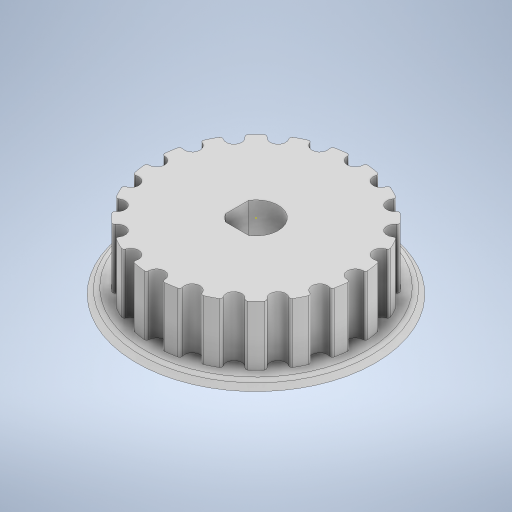
# Autodesk Inventor part: MuftaForRemenSmall
Saved by Autodesk Inventor 2024 (Build 280153000, 153)
## iProperties
Created: 2023-11-07
Part Number: MuftaForRemenSmall
Material: Generic
Document SubType Name: Modeling
Designer: KirikDK
Density: 1 g/cm^3
Appearance: Default
Author: KirikDK
Autodesk Inventor part; units mm, degrees
ref_plane "YZ Plane" through (0, 0, 0) normal (1, 0, 0) x (0, 1, 0)
ref_plane "XZ Plane" through (0, 0, 0) normal (0, 1, 0) x (-1, 0, 0)
ref_plane "XY Plane" through (0, 0, 0) normal (0, 0, 1) x (1, 0, 0)
sketch "Sketch1" plane through (0, 0, 0) normal (0, 1, 0) x (-1, 0, 0)
  circle A0 centre (0, 0) radius 32.5
  dimension "d0" = 65
  constraints: 1 centre point, 1 coincident
  measures "d0" diameter of A0
extrude "Extrusion1" add sketch "Sketch1" along normal blind 21
sketch "Sketch2" plane through (0, 0, 0) normal (0, -1, 0) x (1, 0, 0)
  circle A0 centre (0, 0) radius 38
  dimension "d5" = 76
  constraints: 1 centre point, 1 coincident
  measures "d5" diameter of A0
extrude "Extrusion2" add sketch "Sketch2" against normal blind 2
chamfer "Chamfer1" distance 2 angle 45 1 edges at (-38, 2, 0)
fillet "Fillet1" radius 2 1 edges at (-36.0001, 2, 0)
sketch "Sketch3" plane through (0, 21, 0) normal (0, 1, 0) x (1, 0, 0)
  circle A0 centre (0, 0) radius 7.05
  line L0 (-6, -10) -> (7, -10)
  line L1 (7, -10) -> (7, -6)
  line L2 (7, -6) -> (-6, -6)
  line L3 (-6, -6) -> (-6, -10)
  line L4 (-11, 8) -> (-6, 8)
  line L5 (-6, 8) -> (-6, -6)
  line L6 (-6, -6) -> (-11, -6)
  line L7 (-11, -6) -> (-11, 8)
  point P0 (0.5, -6)
  point P1 (-3.7017, -6)
  point P2 (3.7017, -6)
  point P3 (-6, 3.7017)
  point P4 (-6, -3.7017)
  dimension "d10" = 14.1
  dimension "d11" = 6
  dimension "d23" = 6
  constraints: 16 end point, 4 parallel, 2 horizontal, 2 perpendicular, 1 centre point, 1 coincident, 1 midpoint
  measures "d10" diameter of A0
  measures "d11" vertical distance of point (0, 0) point (0.5, -6)
  measures "d23" distance from line of L5 point (0, 0)
extrude "Extrusion3" cut sketch "Sketch3" against normal blind 40 contours A0 L2 L5 picked at (1.0221, 0.7586)
sketch "Sketch4" plane through (0, 21, 0) normal (0, 1, 0) x (1, 0, 0)
  circle A0 centre (0, 31.6) radius 2.5
  point P0 (0, 0)
  dimension "d14" = 5
  dimension "d15" = 31.6
  constraints: 1 centre point
  measures "d14" diameter of A0
  measures "d15" distance of A0.centre point (0, 0)
extrude "Extrusion4" cut sketch "Sketch4" against normal blind 19
pattern_circular "Circular Pattern1" count 20 over 360 about axis through (0, 21, 0) along (0, -1, 0) of "Extrusion4"
fillet "Fillet2" radius 0.7 42 edges at (-3.7017, 10.5, 6) (3.7017, 10.5, 6) (-2.3638, 11.5, -32.4139) (2.3638, 11.5, -32.4139) (31.5579, 11.5, 7.7684) (32.4139, 11.5, 2.3638) (32.4139, 11.5, -2.3638) (31.5579, 11.5, -7.7684) (30.097, 11.5, -12.2646) (30.097, 11.5, 12.2646) (7.7684, 11.5, -31.5579) (12.2646, 11.5, -30.097) (17.1401, 11.5, -27.6128) (20.9648, 11.5, -24.834) (24.834, 11.5, -20.9648) (27.6128, 11.5, -17.1401) (27.6128, 11.5, 17.1401) (24.834, 11.5, 20.9648) (20.9648, 11.5, 24.834) (17.1401, 11.5, 27.6128) (12.2646, 11.5, 30.097) (7.7684, 11.5, 31.5579) (2.3638, 11.5, 32.4139) (-2.3638, 11.5, 32.4139) (-7.7684, 11.5, 31.5579) (-12.2646, 11.5, 30.097) (-17.1401, 11.5, 27.6128) (-20.9648, 11.5, 24.834) (-30.097, 11.5, -12.2646) (-27.6128, 11.5, -17.1401) (-12.2646, 11.5, -30.097) (-17.1401, 11.5, -27.6128) (-20.9648, 11.5, -24.834) (-24.834, 11.5, -20.9648) (-7.7684, 11.5, -31.5579) (-31.5579, 11.5, -7.7684) (-32.4139, 11.5, -2.3638) (-32.4139, 11.5, 2.3638) (-31.5579, 11.5, 7.7684) (-30.097, 11.5, 12.2646) (-27.6128, 11.5, 17.1401) (-24.834, 11.5, 20.9648)
sketch "Sketch5" plane through (0, 21, 0) normal (0, 1, 0) x (1, 0, 0)
  point P0 (0, 0)
body "Solid1"
